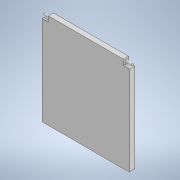
# Autodesk Inventor part: tapa
Saved by Autodesk Inventor 2021 (Build 250183000, 183)
## iProperties
Created: 2022-02-10
Part Number: tapa
Material: Genérico
Document SubType Name: Modeling
Designer: Emanuel
Density: 1 g/cm^3
Appearance: Valor por defecto
Author: Emanuel
Autodesk Inventor part; units mm, degrees
ref_plane "YZ Plane" through (0, 0, 0) normal (1, 0, 0) x (0, 1, 0)
ref_plane "XZ Plane" through (0, 0, 0) normal (0, 1, 0) x (-1, 0, 0)
ref_plane "XY Plane" through (0, 0, 0) normal (0, 0, 1) x (1, 0, 0)
sketch "Boceto1" plane through (0, 0, 0) normal (0, 0, 1) x (1, 0, 0)
  line L0 (-160.5, 235) -> (210.5, 235)
  line L1 (242.5, 208) -> (242.5, -230)
  line L2 (237.5, -235) -> (-187.5, -235)
  line L3 (-192.5, -230) -> (-192.5, 208)
  line L4 (-160.5, 235) -> (-160.5, 208)
  line L5 (-160.5, 208) -> (-192.5, 208)
  line L6 (210.5, 235) -> (210.5, 208)
  line L7 (210.5, 208) -> (242.5, 208)
  arc A0 (-192.5, -230) -> (-187.5, -235) centre (-187.5, -230) ccw
  arc A1 (237.5, -235) -> (242.5, -230) centre (237.5, -230) ccw
  point P0 (0, 0)
  point P1 (242.5, -235)
  point P2 (-192.5, -235)
  dimension "d0" = 435
  dimension "d2" = 32
  dimension "d3" = 27
  dimension "d4" = 32
  dimension "d18" = 5
  constraints: 16 end point, 4 point on circle, 4 point on line, 4 tangent, 2 centre point, 2 parallel, 1 equal radius, 1 horizontal, 1 perpendicular
  measures "d0" distance of point (242.5, -235) point (-192.5, -235)
  measures "d2" distance of L3.end L4.end
  measures "d3" distance of L0.start L4.end
  measures "d4" distance of L1.start L6.end
  measures "d18" radius of A0
extrude "Extrusión1" add sketch "Boceto1" along normal blind 25
sketch "Boceto2" plane through (210.5, 208, 0) normal (1, 0, 0) x (0, 0, -1)
  line L0 (0, 0) -> (-25, 0) projected
  circle A0 centre (-12.5, 13.5) radius 5
  point P0 (0, -208)
  dimension "d7" = 10
  constraints: 1 centre point
  measures "d7" diameter of A0
extrude "Extrusión2" add sketch "Boceto2" along normal blind 32 and the other way blind 403
sketch "Boceto3" plane through (0, 0, 0) normal (0, 0, -1) x (-1, 0, 0)
  line L0 (-21.5, 10) -> (21.5, 10)
  line L1 (21.5, 10) -> (21.5, -10)
  line L2 (21.5, -10) -> (-21.5, -10)
  line L3 (-21.5, -10) -> (-21.5, 10)
  line L4 (-21.5, 10) -> (21.5, -10) construction
  line L5 (21.5, 10) -> (-21.5, -10) construction
  line L6 (24, 12.5) -> (-24, 12.5)
  line L7 (-24, 12.5) -> (-24, -12.5)
  line L8 (-24, -12.5) -> (24, -12.5)
  line L9 (24, -12.5) -> (24, 12.5)
  line L10 (24, 12.5) -> (-24, -12.5) construction
  line L11 (-24, 12.5) -> (24, -12.5) construction
  point P0 (0, 0)
  dimension "d14" = 48
  dimension "d15" = 25
  constraints: 24 end point, 4 midpoint, 4 parallel, 2 horizontal, 2 perpendicular
  measures "d14" distance of L8.end L7.end
  measures "d15" distance of L7.end L6.end
extrude "Extrusión3" add sketch "Boceto3" along normal blind 15
